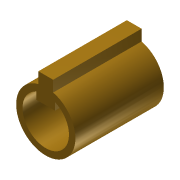
# Autodesk Inventor part: PG71 Adapter
Saved by Autodesk Inventor 2011 (Build 150239000, 239)
## iProperties
Created: 2012-05-18
Part Number: PG71 Adapter
Document SubType Name: Modeling
Designer: dolindner
Density: 8.47 g/cm^3
Material: Brass, Soft Yellow
Mass: 10.2847 g
Surface Area: 16.3724 cm^2
Volume: 1.21425 cm^3
Author: dolindner
Autodesk Inventor part; units mm, degrees
ref_plane "YZ Plane" through (0, 0, 0) normal (1, 0, 0) x (0, 1, 0)
ref_plane "XZ Plane" through (0, 0, 0) normal (0, 1, 0) x (-1, 0, 0)
ref_plane "XY Plane" through (0, 0, 0) normal (0, 0, 1) x (1, 0, 0)
sketch "Sketch1" plane through (0, 0, 0) normal (0, 0, 1) x (1, 0, 0)
  arc A0 (-1.5875, -10.0999) -> (1.5875, -10.0999) centre (0, -16.2745) ccw
  line L0 (-1.5875, -10.0999) -> (-1.5875, -7.7187)
  line L1 (-1.5875, -7.7187) -> (1.5875, -7.7187)
  line L2 (1.5875, -7.7187) -> (1.5875, -10.0999)
  arc A1 (5.0716, -2.4388) -> (6.1971, -2.905) centre (6.228, -1.2388) ccw
  arc A2 (5.0716, -2.4388) -> (0.6091, -1.5512) centre (0, -16.2745) ccw
  arc A3 (-0.6091, -1.5512) -> (0.6091, -1.5512) centre (0, 0) ccw
  arc A4 (-0.6091, -1.5512) -> (-5.0716, -2.4388) centre (0, -16.2745) ccw
  arc A5 (-6.1971, -2.905) -> (-5.0716, -2.4388) centre (-6.228, -1.2388) ccw
  arc A6 (-6.1971, -2.905) -> (-9.9802, -5.4328) centre (0, -16.2745) ccw
  arc A7 (-10.8417, -6.2943) -> (-9.9802, -5.4328) centre (-11.5078, -4.7667) ccw
  arc A8 (-10.8417, -6.2943) -> (-13.3695, -10.0774) centre (0, -16.2745) ccw
  arc A9 (-13.8357, -11.2029) -> (-13.3695, -10.0774) centre (-15.0357, -10.0465) ccw
  arc A10 (-13.8357, -11.2029) -> (-14.7233, -15.6654) centre (0, -16.2745) ccw
  arc A11 (-14.7233, -16.8837) -> (-14.7233, -15.6654) centre (-16.2745, -16.2745) ccw
  arc A12 (-14.7233, -16.8837) -> (-13.8357, -21.3461) centre (0, -16.2745) ccw
  arc A13 (-13.3695, -22.4717) -> (-13.8357, -21.3461) centre (-15.0357, -22.5025) ccw
  arc A14 (-13.3695, -22.4717) -> (-10.8417, -26.2548) centre (0, -16.2745) ccw
  arc A15 (-9.9802, -27.1162) -> (-10.8417, -26.2548) centre (-11.5078, -27.7823) ccw
  arc A16 (-9.9802, -27.1162) -> (-6.1971, -29.644) centre (0, -16.2745) ccw
  arc A17 (-5.0716, -30.1102) -> (-6.1971, -29.644) centre (-6.228, -31.3102) ccw
  arc A18 (-5.0716, -30.1102) -> (-0.6091, -30.9978) centre (0, -16.2745) ccw
  arc A19 (0.6091, -30.9978) -> (-0.6091, -30.9978) centre (0, -32.549) ccw
  arc A20 (0.6091, -30.9978) -> (5.0716, -30.1102) centre (0, -16.2745) ccw
  arc A21 (6.1971, -29.644) -> (5.0716, -30.1102) centre (6.228, -31.3102) ccw
  arc A22 (6.1971, -29.644) -> (9.9802, -27.1162) centre (0, -16.2745) ccw
  arc A23 (10.8417, -26.2548) -> (9.9802, -27.1162) centre (11.5078, -27.7823) ccw
  arc A24 (10.8417, -26.2548) -> (13.3695, -22.4717) centre (0, -16.2745) ccw
  arc A25 (13.8357, -21.3461) -> (13.3695, -22.4717) centre (15.0357, -22.5025) ccw
  arc A26 (13.8357, -21.3461) -> (14.7233, -16.8837) centre (0, -16.2745) ccw
  arc A27 (14.7233, -15.6654) -> (14.7233, -16.8837) centre (16.2745, -16.2745) ccw
  arc A28 (14.7233, -15.6654) -> (13.8357, -11.2029) centre (0, -16.2745) ccw
  arc A29 (13.3695, -10.0774) -> (13.8357, -11.2029) centre (15.0357, -10.0465) ccw
  arc A30 (13.3695, -10.0774) -> (10.8417, -6.2943) centre (0, -16.2745) ccw
  arc A31 (9.9802, -5.4328) -> (10.8417, -6.2943) centre (11.5078, -4.7667) ccw
  arc A32 (9.9802, -5.4328) -> (6.1971, -2.905) centre (0, -16.2745) ccw
  line L3 (-2, -13.2745) -> (-2, -11.6919)
  arc A33 (-2, -11.6919) -> (2, -11.6919) centre (0, -16.2745) ccw
  line L4 (2, -13.2745) -> (2, -11.6919)
  line L5 (-2, -13.2745) -> (2, -13.2745)
  constraints: 66 point on circle, 33 centre point, 6 end point
extrude "Extrusion1" add sketch "Sketch1" along normal blind 19.05 contours L0 L1 L2 A0
body "Solid1"
